Autodesk Fusion 360 part; units mm, degrees
note: some values were not read from the file. Set by a fixed rule: which sketch regions a step uses.
(part 3 of 6)
  line L1897 (389.5, 225.3453) -> (391.5, 224.1906)
  line L1898 (364.75, 196.4178) -> (364.75, 194.1084)
  line L1899 (377.75, 201.9537) -> (379.75, 203.1084)
  line L1900 (381.25, 203.1084) -> (383.25, 201.9537)
  line L1901 (386.75, 230.1084) -> (388.75, 228.9537)
  line L1902 (355, 207.3453) -> (355, 209.6547)
  line L1903 (381.25, 205.4178) -> (381.25, 203.1084)
  line L1904 (366.75, 197.5725) -> (364.75, 196.4178)
  line L1905 (399.75, 237.9537) -> (401.75, 239.1084)
  line L1906 (363.25, 212.1084) -> (363.25, 214.4178)
  line L1907 (390.75, 221.1084) -> (390.75, 223.4178)
  line L1908 (377, 198.3453) -> (377, 200.6547)
  line L1909 (369.5, 233.1906) -> (371.5, 234.3453)
  line L1910 (361.25, 206.5725) -> (359.25, 205.4178)
  line L1911 (388, 225.3453) -> (388, 227.6547)
  line L1912 (362, 198.3453) -> (364, 197.1906)
  line L1913 (368.75, 194.1084) -> (368.75, 196.4178)
  line L1914 (385.25, 221.1084) -> (385.25, 223.4178)
  line L1915 (364.75, 214.4178) -> (364.75, 212.1084)
  line L1916 (389.5, 225.3453) -> (391.5, 224.1906)
  line L1917 (371.5, 227.6547) -> (369.5, 228.8094)
  line L1918 (356.5, 207.3453) -> (358.5, 206.1906)
  line L1919 (366, 191.6547) -> (364, 192.8094)
  line L1920 (364.75, 203.1084) -> (366.75, 201.9537)
  line L1921 (364, 197.1906) -> (366, 198.3453)
  line L1922 (399, 234.3453) -> (399, 236.6547)
  line L1923 (353.75, 212.1084) -> (355.75, 210.9537)
  line L1924 (358.5, 210.8094) -> (356.5, 209.6547)
  line L1925 (366, 200.6547) -> (364, 201.8094)
  line L1926 (393.5, 234.3453) -> (393.5, 236.6547)
  line L1927 (358.5, 206.1906) -> (360.5, 207.3453)
  line L1928 (384, 225.3453) -> (386, 224.1906)
  line L1929 (364.75, 194.1084) -> (366.75, 192.9537)
  line L1930 (371.5, 236.6547) -> (369.5, 237.8094)
  line L1931 (381.25, 241.4178) -> (381.25, 239.1084)
  line L1932 (357.75, 205.4178) -> (355.75, 206.5725)
  line L1933 (373, 252.3453) -> (375, 251.1906)
  line L1934 (381.25, 196.4178) -> (381.25, 194.1084)
  line L1935 (364, 192.8094) -> (362, 191.6547)
  line L1936 (372.25, 251.5725) -> (370.25, 250.4178)
  line L1937 (355.75, 210.9537) -> (357.75, 212.1084)
  line L1938 (372.25, 242.5725) -> (370.25, 241.4178)
  line L1939 (380.5, 201.8094) -> (378.5, 200.6547)
  line L1940 (393.5, 234.3453) -> (393.5, 236.6547)
  line L1941 (369.5, 242.1906) -> (371.5, 243.3453)
  line L1942 (392.25, 241.4178) -> (392.25, 239.1084)
  line L1943 (372.25, 251.5725) -> (370.25, 250.4178)
  line L1944 (357.75, 221.1084) -> (357.75, 223.4178)
  line L1945 (386.75, 223.4178) -> (386.75, 221.1084)
  line L1946 (388.75, 224.5725) -> (386.75, 223.4178)
  line L1947 (366, 198.3453) -> (366, 200.6547)
  line L1948 (355.75, 210.9537) -> (357.75, 212.1084)
  line L1949 (375.75, 203.1084) -> (377.75, 201.9537)
  line L1950 (368.75, 196.4178) -> (366.75, 197.5725)
  line L1951 (386, 228.8094) -> (384, 227.6547)
  line L1952 (384, 227.6547) -> (384, 225.3453)
  line L1953 (383.25, 215.5725) -> (381.25, 214.4178)
  line L1954 (390.75, 223.4178) -> (388.75, 224.5725)
  line L1955 (375, 237.8094) -> (373, 236.6547)
  line L1956 (381.25, 194.1084) -> (383.25, 192.9537)
  line L1957 (357.75, 205.4178) -> (355.75, 206.5725)
  line L1958 (402.5, 237.8094) -> (400.5, 236.6547)
  line L1959 (374.25, 248.1084) -> (374.25, 250.4178)
  line L1960 (371.5, 236.6547) -> (369.5, 237.8094)
  line L1961 (356.5, 209.6547) -> (356.5, 207.3453)
  line L1962 (380.5, 197.1906) -> (382.5, 198.3453)
  line L1963 (379.75, 194.1084) -> (379.75, 196.4178)
  line L1964 (370.25, 241.4178) -> (370.25, 239.1084)
  line L1965 (404.5, 227.6547) -> (402.5, 228.8094)
  line L1966 (400.5, 236.6547) -> (400.5, 234.3453)
  line L1967 (402.5, 237.8094) -> (400.5, 236.6547)
  line L1968 (371.5, 243.3453) -> (371.5, 245.6547)
  line L1969 (356.5, 209.6547) -> (356.5, 207.3453)
  line L1970 (382.5, 198.3453) -> (382.5, 200.6547)
  line L1971 (362, 198.3453) -> (364, 197.1906)
  line L1972 (381.25, 196.4178) -> (381.25, 194.1084)
  line L1973 (386, 224.1906) -> (388, 225.3453)
  line L1974 (395, 236.6547) -> (395, 234.3453)
  line L1975 (382.5, 200.6547) -> (380.5, 201.8094)
  line L1976 (355.75, 206.5725) -> (353.75, 205.4178)
  line L1977 (377.75, 192.9537) -> (379.75, 194.1084)
  line L1978 (353.75, 223.4178) -> (353.75, 221.1084)
  line L1979 (364.75, 194.1084) -> (366.75, 192.9537)
  line L1980 (389.5, 227.6547) -> (389.5, 225.3453)
  line L1981 (400.5, 234.3453) -> (402.5, 233.1906)
  line L1982 (400.5, 236.6547) -> (400.5, 234.3453)
  line L1983 (374.25, 241.4178) -> (372.25, 242.5725)
  line L1984 (381.25, 212.1084) -> (383.25, 210.9537)
  line L1985 (370.25, 250.4178) -> (370.25, 248.1084)
  line L1986 (369.5, 233.1906) -> (371.5, 234.3453)
  line L1987 (395, 236.6547) -> (395, 234.3453)
  line L1988 (375.75, 194.1084) -> (377.75, 192.9537)
  line L1989 (383.25, 206.5725) -> (381.25, 205.4178)
  line L1990 (352.25, 221.1084) -> (352.25, 223.4178)
  line L1991 (346.75, 221.1084) -> (346.75, 223.4178)
  line L1992 (375.75, 241.4178) -> (375.75, 239.1084)
  line L1993 (346.75, 221.1084) -> (346.75, 223.4178)
  line L1994 (370.25, 250.4178) -> (370.25, 248.1084)
  line L1995 (356.5, 216.3453) -> (358.5, 215.1906)
  line L1996 (378.5, 200.6547) -> (378.5, 198.3453)
  line L1997 (385.25, 205.4178) -> (383.25, 206.5725)
  line L1998 (370.25, 248.1084) -> (372.25, 246.9537)
  line L1999 (372.25, 246.9537) -> (374.25, 248.1084)
  line L2000 (369.5, 251.1906) -> (371.4564, 252.3202)
  line L2001 (388.75, 206.5725) -> (386.75, 205.4178)
  line L2002 (379.75, 196.4178) -> (377.75, 197.5725)
  line L2003 (390.75, 205.4178) -> (388.75, 206.5725)
  line L2004 (375, 237.8094) -> (373, 236.6547)
  line L2005 (353, 215.1906) -> (355, 216.3453)
  line L2006 (348.25, 223.4178) -> (348.25, 221.1084)
  line L2007 (386, 210.8094) -> (384, 209.6547)
  line L2008 (372.25, 237.9537) -> (374.25, 239.1084)
  line L2009 (355, 218.6547) -> (353, 219.8094)
  line L2010 (371.5, 218.6547) -> (369.5, 219.8094)
  line L2011 (384, 209.6547) -> (384, 207.3453)
  line L2012 (369.5, 251.1906) -> (371.4564, 252.3202)
  line L2013 (385.25, 196.4178) -> (383.25, 197.5725)
  line L2014 (361.25, 215.5725) -> (359.25, 214.4178)
  line L2015 (381.25, 203.1084) -> (383.25, 201.9537)
  line L2016 (375, 246.8094) -> (373, 245.6547)
  line L2017 (372.25, 237.9537) -> (374.25, 239.1084)
  line L2018 (374.25, 239.1084) -> (374.25, 241.4178)
  line L2019 (355.75, 215.5725) -> (353.75, 214.4178)
  line L2020 (383.25, 201.9537) -> (385.25, 203.1084)
  line L2021 (385.25, 214.4178) -> (383.25, 215.5725)
  line L2022 (381.25, 194.1084) -> (383.25, 192.9537)
  line L2023 (380.5, 201.8094) -> (378.5, 200.6547)
  line L2024 (382.5, 225.3453) -> (382.5, 227.6547)
  line L2025 (352.25, 239.1084) -> (352.25, 241.4178)
  line L2026 (357.75, 214.4178) -> (355.75, 215.5725)
  line L2027 (389.5, 209.6547) -> (389.5, 207.3453)
  line L2028 (370.25, 248.1084) -> (372.25, 246.9537)
  line L2029 (373, 252.4428) -> (373, 252.3453)
  line L2030 (385.25, 214.4178) -> (383.25, 215.5725)
  line L2031 (375.75, 194.1084) -> (377.75, 192.9537)
  line L2032 (383.25, 210.9537) -> (385.25, 212.1084)
  line L2033 (386.75, 212.1084) -> (388.75, 210.9537)
  line L2034 (383.25, 206.5725) -> (381.25, 205.4178)
  line L2035 (388, 207.3453) -> (388, 209.6547)
  line L2036 (382.5, 198.3453) -> (382.5, 200.6547)
  line L2037 (375.75, 223.4178) -> (375.75, 221.1084)
  line L2038 (383.25, 197.5725) -> (381.25, 196.4178)
  line L2039 (383.25, 197.5725) -> (381.25, 196.4178)
  line L2040 (377.75, 228.9537) -> (379.75, 230.1084)
  line L2041 (381.25, 223.4178) -> (381.25, 221.1084)
  line L2042 (383.25, 192.9537) -> (385.25, 194.1084)
  line L2043 (377.75, 197.5725) -> (375.75, 196.4178)
  line L2044 (381.25, 212.1084) -> (383.25, 210.9537)
  line L2045 (355, 216.3453) -> (355, 218.6547)
  line L2046 (383.25, 210.9537) -> (385.25, 212.1084)
  line L2047 (359.25, 223.4178) -> (359.25, 221.1084)
  line L2048 (388, 207.3453) -> (388, 209.6547)
  line L2049 (353, 215.1906) -> (355, 216.3453)
  line L2050 (360.5, 218.6547) -> (358.5, 219.8094)
  line L2051 (390.75, 205.4178) -> (388.75, 206.5725)
  arc A62 (371.4564, 252.3202) -> (368.3398, 251.8605) centre (375, 217.5) ccw
  line L2052 (388, 209.6547) -> (386, 210.8094)
  line L2053 (369.5, 224.1906) -> (371.5, 225.3453)
  line L2054 (373, 245.6547) -> (373, 243.3453)
  line L2055 (380.5, 197.1906) -> (382.5, 198.3453)
  line L2056 (382.5, 225.3453) -> (382.5, 227.6547)
  line L2057 (389.5, 209.6547) -> (389.5, 207.3453)
  line L2058 (373, 243.3453) -> (375, 242.1906)
  line L2059 (383.25, 192.9537) -> (385.25, 194.1084)
  line L2060 (358.5, 219.8094) -> (356.5, 218.6547)
  line L2061 (360.5, 216.3453) -> (360.5, 218.6547)
  line L2062 (358.5, 215.1906) -> (360.5, 216.3453)
  line L2063 (370.25, 239.1084) -> (372.25, 237.9537)
  line L2064 (375.75, 223.4178) -> (375.75, 221.1084)
  line L2065 (371.5, 243.3453) -> (371.5, 245.6547)
  line L2066 (389.5, 207.3453) -> (391.5, 206.1906)
  line L2067 (375.75, 230.1084) -> (377.75, 228.9537)
  line L2068 (388.75, 210.9537) -> (390.75, 212.1084)
  line L2069 (386, 206.1906) -> (388, 207.3453)
  line L2070 (379.75, 221.1084) -> (379.75, 223.4178)
  line L2071 (378.5, 227.6547) -> (378.5, 225.3453)
  line L2072 (374.25, 248.1084) -> (374.25, 250.4178)
  line L2073 (386.75, 232.4178) -> (386.75, 230.1084)
  line L2074 (389.5, 207.3453) -> (391.5, 206.1906)
  line L2075 (370.25, 239.1084) -> (372.25, 237.9537)
  line L2076 (362, 218.6547) -> (362, 216.3453)
  line L2077 (384, 209.6547) -> (384, 207.3453)
  line L2078 (360.5, 218.6547) -> (358.5, 219.8094)
  line L2079 (379.75, 248.1084) -> (379.75, 250.4178)
  line L2080 (369.5, 215.1906) -> (371.5, 216.3453)
  line L2081 (358.5, 219.8094) -> (356.5, 218.6547)
  line L2082 (377, 225.3453) -> (377, 227.6547)
  line L2083 (388.75, 206.5725) -> (386.75, 205.4178)
  line L2084 (360.5, 225.3453) -> (360.5, 227.6547)
  line L2085 (391.5, 210.8094) -> (389.5, 209.6547)
  line L2086 (383.25, 215.5725) -> (381.25, 214.4178)
  line L2087 (372.25, 246.9537) -> (374.25, 248.1084)
  line L2088 (371.5, 227.6547) -> (369.5, 228.8094)
  line L2089 (355, 209.6547) -> (353, 210.8094)
  line L2090 (359.25, 241.4178) -> (359.25, 239.1084)
  line L2091 (391.5, 210.8094) -> (389.5, 209.6547)
  line L2092 (374.25, 250.4178) -> (372.25, 251.5725)
  line L2093 (377.75, 224.5725) -> (375.75, 223.4178)
  line L2094 (386, 206.1906) -> (388, 207.3453)
  line L2095 (348.25, 240.0707) -> (348.25, 239.1084)
  line L2096 (374.25, 239.1084) -> (374.25, 241.4178)
  line L2097 (381.25, 223.4178) -> (381.25, 221.1084)
  line L2098 (385.25, 205.4178) -> (383.25, 206.5725)
  line L2099 (373, 252.4428) -> (373, 252.3453)
  line L2100 (380.5, 224.1906) -> (382.5, 225.3453)
  line L2101 (355.75, 228.9537) -> (357.75, 230.1084)
  line L2102 (382.5, 227.6547) -> (380.5, 228.8094)
  line L2103 (355.75, 215.5725) -> (353.75, 214.4178)
  line L2104 (369.5, 242.1906) -> (371.5, 243.3453)
  line L2105 (371.5, 218.6547) -> (369.5, 219.8094)
  line L2106 (369.5, 215.1906) -> (371.5, 216.3453)
  line L2107 (353.75, 221.1084) -> (355.75, 219.9537)
  line L2108 (373, 243.3453) -> (375, 242.1906)
  line L2109 (379.75, 221.1084) -> (379.75, 223.4178)
  line L2110 (357.75, 239.1084) -> (357.75, 241.4178)
  line L2111 (358.5, 215.1906) -> (360.5, 216.3453)
  line L2112 (383.25, 201.9537) -> (385.25, 203.1084)
  line L2113 (390.75, 212.1084) -> (390.75, 214.4178)
  line L2114 (385.25, 196.4178) -> (383.25, 197.5725)
  line L2115 (373, 245.6547) -> (373, 243.3453)
  line L2116 (356.5, 227.6547) -> (356.5, 225.3453)
  line L2117 (353, 206.1906) -> (355, 207.3453)
  line L2118 (355, 216.3453) -> (355, 218.6547)
  line L2119 (384, 207.3453) -> (386, 206.1906)
  line L2120 (377, 225.3453) -> (377, 227.6547)
  line L2121 (382.5, 209.6547) -> (380.5, 210.8094)
  line L2122 (388, 209.6547) -> (386, 210.8094)
  line L2123 (373, 236.6547) -> (373, 234.3453)
  line L2124 (388, 245.6547) -> (386, 246.8094)
  line L2125 (360.5, 216.3453) -> (360.5, 218.6547)
  line L2126 (372.25, 242.5725) -> (370.25, 241.4178)
  line L2127 (379.75, 230.1084) -> (379.75, 232.4178)
  line L2128 (359.25, 221.1084) -> (361.25, 219.9537)
  line L2129 (357.75, 223.4178) -> (355.75, 224.5725)
  line L2130 (392.25, 214.4178) -> (392.25, 212.1084)
  line L2131 (375, 246.8094) -> (373, 245.6547)
  line L2132 (356.5, 225.3453) -> (358.5, 224.1906)
  line L2133 (362, 227.6547) -> (362, 225.3453)
  line L2134 (373, 252.3453) -> (375, 251.1906)
  line L2135 (362, 227.6547) -> (362, 225.3453)
  line L2136 (355.75, 219.9537) -> (357.75, 221.1084)
  line L2137 (375.75, 230.1084) -> (377.75, 228.9537)
  line L2138 (378.5, 207.3453) -> (380.5, 206.1906)
  line L2139 (356.5, 225.3453) -> (358.5, 224.1906)
  line L2140 (382.5, 209.6547) -> (380.5, 210.8094)
  line L2141 (386, 210.8094) -> (384, 209.6547)
  line L2142 (359.25, 230.1084) -> (361.25, 228.9537)
  line L2143 (392.25, 214.4178) -> (392.25, 212.1084)
  line L2144 (384, 207.3453) -> (386, 206.1906)
  line L2145 (386.75, 248.1084) -> (388.75, 246.9537)
  line L2146 (378.5, 225.3453) -> (380.5, 224.1906)
  line L2147 (359.25, 230.1084) -> (361.25, 228.9537)
  line L2148 (385.25, 212.1084) -> (385.25, 214.4178)
  line L2149 (386, 246.8094) -> (384, 245.6547)
  line L2150 (377, 207.3453) -> (377, 209.6547)
  line L2151 (371.5, 234.3453) -> (371.5, 236.6547)
  line L2152 (380.5, 224.1906) -> (382.5, 225.3453)
  line L2153 (379.75, 223.4178) -> (377.75, 224.5725)
  line L2154 (374.25, 250.4178) -> (372.25, 251.5725)
  line L2155 (357.75, 214.4178) -> (355.75, 215.5725)
  line L2156 (379.75, 230.1084) -> (379.75, 232.4178)
  line L2157 (359.25, 221.1084) -> (361.25, 219.9537)
  line L2158 (386.75, 212.1084) -> (388.75, 210.9537)
  line L2159 (361.25, 224.5725) -> (359.25, 223.4178)
  line L2160 (389.5, 243.3453) -> (391.5, 242.1906)
  line L2161 (380.5, 228.8094) -> (378.5, 227.6547)
  line L2162 (357.75, 223.4178) -> (355.75, 224.5725)
  line L2163 (390.75, 212.1084) -> (390.75, 214.4178)
  line L2164 (361.25, 215.5725) -> (359.25, 214.4178)
  line L2165 (375.75, 250.4178) -> (375.75, 248.1084)
  line L2166 (374.25, 241.4178) -> (372.25, 242.5725)
  line L2167 (375.75, 212.1084) -> (377.75, 210.9537)
  line L2168 (370.25, 241.4178) -> (370.25, 239.1084)
  line L2169 (382.5, 227.6547) -> (380.5, 228.8094)
  line L2170 (377.75, 228.9537) -> (379.75, 230.1084)
  line L2171 (388.75, 210.9537) -> (390.75, 212.1084)
  line L2172 (356.5, 218.6547) -> (356.5, 216.3453)
  line L2173 (362, 218.6547) -> (362, 216.3453)
  line L2174 (373, 236.6547) -> (373, 234.3453)
  line L2175 (377.75, 206.5725) -> (375.75, 205.4178)
  line L2176 (379.75, 223.4178) -> (377.75, 224.5725)
  line L2177 (378.5, 225.3453) -> (380.5, 224.1906)
  line L2178 (356.5, 218.6547) -> (356.5, 216.3453)
  line L2179 (361.25, 224.5725) -> (359.25, 223.4178)
  arc A63 (371.4564, 252.3202) -> (368.3398, 251.8605) centre (375, 217.5) ccw
  line L2180 (379.75, 205.4178) -> (377.75, 206.5725)
  line L2181 (380.5, 228.8094) -> (378.5, 227.6547)
  line L2182 (355.75, 219.9537) -> (357.75, 221.1084)
  line L2183 (360.5, 227.6547) -> (358.5, 228.8094)
  line L2184 (377.75, 224.5725) -> (375.75, 223.4178)
  line L2185 (382.5, 207.3453) -> (382.5, 209.6547)
  line L2186 (353.75, 241.4178) -> (353.75, 239.1084)
  line L2187 (356.5, 216.3453) -> (358.5, 215.1906)
  line L2188 (388.75, 242.5725) -> (386.75, 241.4178)
  line L2189 (389.5, 245.6547) -> (389.5, 243.3453)
  line L2190 (371.5, 234.3453) -> (371.5, 236.6547)
  line L2191 (353.75, 230.1084) -> (355.75, 228.9537)
  arc A64 (387.3612, 184.7555) -> (390.75, 186.244) centre (375, 217.5) ccw
  arc A65 (387.3612, 184.7555) -> (390.75, 186.244) centre (375, 217.5) ccw
  line L2192 (388.75, 188.5725) -> (386.75, 187.4178)
  line L2193 (390.75, 187.4178) -> (388.75, 188.5725)
  line L2194 (384, 189.3453) -> (386, 188.1906)
  line L2195 (388, 189.3453) -> (388, 191.6547)
  line L2196 (380.5, 188.1906) -> (382.5, 189.3453)
  line L2197 (381.25, 187.4178) -> (381.25, 185.1084)
  line L2198 (386.75, 187.4178) -> (386.75, 185.1084)
  line L2199 (380.5, 188.1906) -> (382.5, 189.3453)
  line L2200 (375.75, 187.4178) -> (375.75, 185.1084)
  line L2201 (386, 188.1906) -> (388, 189.3453)
  line L2202 (379.75, 187.4178) -> (377.75, 188.5725)
  line L2203 (379.75, 185.1084) -> (379.75, 187.4178)
  line L2204 (386.75, 187.4178) -> (386.75, 185.1084)
  line L2205 (375.75, 187.4178) -> (375.75, 185.1084)
  line L2206 (381.25, 187.4178) -> (381.25, 185.1084)
  line L2207 (388.75, 188.5725) -> (386.75, 187.4178)
  line L2208 (379.75, 185.1084) -> (379.75, 187.4178)
  line L2209 (385.25, 185.1084) -> (385.25, 187.4178)
  line L2210 (375, 233.1906) -> (377, 234.3453)
  line L2211 (390.75, 187.4178) -> (388.75, 188.5725)
  line L2212 (385.25, 185.1084) -> (385.25, 187.4178)
  line L2213 (402.5, 197.1906) -> (404.1665, 198.1527)
  line L2214 (400.5, 198.3453) -> (402.5, 197.1906)
  line L2215 (404.5, 200.6547) -> (402.5, 201.8094)
  line L2216 (402.5, 206.1906) -> (404.5, 207.3453)
  line L2217 (400.5, 198.3453) -> (402.5, 197.1906)
  line L2218 (402.5, 201.8094) -> (400.5, 200.6547)
  line L2219 (404.5, 200.6547) -> (402.5, 201.8094)
  line L2220 (400.5, 207.3453) -> (402.5, 206.1906)
  line L2221 (395, 200.6547) -> (395, 198.3453)
  line L2222 (399, 198.3453) -> (399, 200.6547)
  line L2223 (395, 200.6547) -> (395, 198.3453)
  line L2224 (393.5, 198.3453) -> (393.5, 200.6547)
  line L2225 (400.5, 200.6547) -> (400.5, 198.3453)
  line L2226 (402.5, 201.8094) -> (400.5, 200.6547)
  line L2227 (393.5, 198.3453) -> (393.5, 200.6547)
  line L2228 (402.5, 206.1906) -> (404.5, 207.3453)
  line L2229 (400.5, 200.6547) -> (400.5, 198.3453)
  line L2230 (391.5, 188.1906) -> (393.5, 189.3453)
  line L2231 (389.5, 189.3453) -> (391.5, 188.1906)
  line L2232 (393.5, 189.3453) -> (393.5, 191.6547)
  line L2233 (390.75, 186.244) -> (390.75, 187.4178)
  line L2234 (393.5, 189.3453) -> (393.5, 191.6547)
  line L2235 (392.25, 187.4178) -> (392.25, 187.0461)
  line L2236 (391.5, 188.1906) -> (393.5, 189.3453)
  line L2237 (390.75, 186.244) -> (390.75, 187.4178)
  line L2238 (389.5, 189.3453) -> (391.5, 188.1906)
  line L2239 (389.5, 191.6547) -> (389.5, 189.3453)
  line L2240 (392.25, 187.4178) -> (392.25, 187.0461)
  line L2241 (399.75, 206.5725) -> (397.75, 205.4178)
  line L2242 (399.75, 201.9537) -> (401.75, 203.1084)
  line L2243 (397, 201.8094) -> (395, 200.6547)
  line L2244 (395, 207.3453) -> (397, 206.1906)
  line L2245 (394.25, 201.9537) -> (396.25, 203.1084)
  line L2246 (395, 207.3453) -> (397, 206.1906)
  line L2247 (397.75, 205.4178) -> (397.75, 203.1084)
  line L2248 (401.75, 203.1084) -> (401.75, 205.4178)
  line L2249 (396.25, 203.1084) -> (396.25, 205.4178)
  line L2250 (397, 206.1906) -> (399, 207.3453)
  line L2251 (401.75, 205.4178) -> (399.75, 206.5725)
  line L2252 (397, 206.1906) -> (399, 207.3453)
  line L2253 (397.75, 205.4178) -> (397.75, 203.1084)
  line L2254 (397.75, 203.1084) -> (399.75, 201.9537)
  line L2255 (397, 201.8094) -> (395, 200.6547)
  line L2256 (399, 198.3453) -> (399, 200.6547)
  line L2257 (399, 200.6547) -> (397, 201.8094)
  line L2258 (399.75, 206.5725) -> (397.75, 205.4178)
  line L2259 (399.75, 201.9537) -> (401.75, 203.1084)
  line L2260 (396.25, 205.4178) -> (394.25, 206.5725)
  line L2261 (394.25, 201.9537) -> (396.25, 203.1084)
  line L2262 (405.25, 206.5725) -> (403.25, 205.4178)
  line L2263 (405.25, 206.5725) -> (403.25, 205.4178)
  line L2264 (403.25, 203.1084) -> (405.25, 201.9537)
  line L2265 (403.25, 205.4178) -> (403.25, 203.1084)
  line L2266 (407.25, 205.4178) -> (405.25, 206.5725)
  arc A66 (406.7807, 202.8375) -> (407.25, 203.9008) centre (375, 217.5) ccw
  arc A67 (406.7807, 202.8375) -> (407.25, 203.9008) centre (375, 217.5) ccw
  line L2267 (405.25, 201.9537) -> (406.7807, 202.8375)
  line L2268 (408, 206.1906) -> (408.1524, 206.2786)
  line L2269 (407.25, 203.9008) -> (407.25, 205.4178)
  arc A68 (404.1665, 198.1527) -> (404.5, 198.6652) centre (375, 217.5) ccw
  line L2270 (403.25, 205.4178) -> (403.25, 203.1084)
  line L2271 (406, 207.3453) -> (408, 206.1906)
  line L2272 (403.25, 203.1084) -> (405.25, 201.9537)
  arc A69 (404.1665, 198.1527) -> (404.5, 198.6652) centre (375, 217.5) ccw
  line L2273 (405.25, 201.9537) -> (406.7807, 202.8375)
  line L2274 (407.25, 205.4178) -> (405.25, 206.5725)
  line L2275 (408, 206.1906) -> (408.1524, 206.2786)
  line L2276 (404.5, 198.6652) -> (404.5, 200.6547)
  line L2277 (406, 207.3453) -> (408, 206.1906)
  line L2278 (404.5, 198.6652) -> (404.5, 200.6547)
  line L2279 (407.25, 203.9008) -> (407.25, 205.4178)
  line L2280 (396.25, -88.5822) -> (394.25, -87.4275)
  line L2281 (397.75, -90.8916) -> (399.75, -92.0463)
  line L2282 (401.75, -90.8916) -> (401.75, -88.5822)
  line L2283 (399, -93.3453) -> (397, -92.1906)
  line L2284 (396.25, -90.8916) -> (396.25, -88.5822)
  line L2285 (401.75, -88.5822) -> (399.75, -87.4275)
  line L2286 (395, -95.6547) -> (397, -96.8094)
  line L2287 (401.75, -97.5822) -> (399.75, -96.4275)
  line L2288 (397.75, -97.5822) -> (397.75, -99.8916)
  line L2289 (397.75, -97.5822) -> (397.75, -99.8916)
  arc A70 (400.2057, -100.7831) -> (401.75, -99.0707) centre (375, -76.5) ccw
  line L2290 (397, -96.8094) -> (399, -95.6547)
  line L2291 (397.75, -99.8916) -> (399.75, -101.0463)
  line L2292 (396.25, -97.5822) -> (394.25, -96.4275)
  line L2293 (396.25, -97.5822) -> (394.25, -96.4275)
  line L2294 (401.75, -99.0707) -> (401.75, -97.5822)
  line L2295 (399.75, -101.0463) -> (400.2057, -100.7831)
  arc A71 (400.2057, -100.7831) -> (401.75, -99.0707) centre (375, -76.5) ccw
  line L2296 (396.25, -99.8916) -> (396.25, -97.5822)
  line L2297 (396.25, -99.8916) -> (396.25, -97.5822)
  line L2298 (401.75, -97.5822) -> (399.75, -96.4275)
  line L2299 (397.75, -99.8916) -> (399.75, -101.0463)
  line L2300 (399.75, -101.0463) -> (400.2057, -100.7831)
  line L2301 (399.75, -96.4275) -> (397.75, -97.5822)
  line L2302 (401.75, -99.0707) -> (401.75, -97.5822)
  line L2303 (395, -95.6547) -> (397, -96.8094)
  line L2304 (399.75, -96.4275) -> (397.75, -97.5822)
  line L2305 (397, -96.8094) -> (399, -95.6547)
  line L2306 (394.25, -101.0463) -> (396.25, -99.8916)
  line L2307 (394.25, -101.0463) -> (396.25, -99.8916)
  line L2308 (375, -105.8094) -> (377, -104.6547)
  line L2309 (389.5, -102.3453) -> (389.5, -104.6547)
  arc A72 (395.442, -104.9099) -> (398.7552, -102.2039) centre (375, -76.5) ccw
  line L2310 (395, -104.6547) -> (395.442, -104.9099)
  line L2311 (395, -102.3453) -> (395, -104.6547)
  arc A73 (395.442, -104.9099) -> (398.7552, -102.2039) centre (375, -76.5) ccw
  line L2312 (395, -102.3453) -> (395, -104.6547)
  line L2313 (395, -104.6547) -> (395.442, -104.9099)
  line L2314 (396.25, -81.8916) -> (396.25, -79.5822)
  line L2315 (397.75, -79.5822) -> (397.75, -81.8916)
  line L2316 (377, -57.3453) -> (375, -56.1906)
  line L2317 (395, -77.6547) -> (397, -78.8094)
  line L2318 (399.75, -83.0463) -> (401.75, -81.8916)
  line L2319 (375, -87.8094) -> (377, -86.6547)
  line L2320 (399, -84.3453) -> (397, -83.1906)
  line L2321 (397.75, -81.8916) -> (399.75, -83.0463)
  line L2322 (399, -84.3453) -> (397, -83.1906)
  line L2323 (397.75, -81.8916) -> (399.75, -83.0463)
  line L2324 (396.25, -79.5822) -> (394.25, -78.4275)
  line L2325 (375, -96.8094) -> (377, -95.6547)
  line L2326 (397.75, -79.5822) -> (397.75, -81.8916)
  line L2327 (375, -87.8094) -> (377, -86.6547)
  line L2328 (401.75, -81.8916) -> (401.75, -79.5822)
  line L2329 (375, -69.8094) -> (377, -68.6547)
  line L2330 (394.25, -83.0463) -> (396.25, -81.8916)
  arc A74 (377, -41.5572) -> (373, -41.5572) centre (375, -76.5) ccw
  line L2331 (375, -78.8094) -> (377, -77.6547)
  line L2332 (377, -84.3453) -> (375, -83.1906)
  line L2333 (375, -60.8094) -> (377, -59.6547)
  line L2334 (399.75, -83.0463) -> (401.75, -81.8916)
  line L2335 (377, -111.3453) -> (375, -110.1906)
  line L2336 (375, -78.8094) -> (377, -77.6547)
  line L2337 (375, -42.8094) -> (377, -41.6547)
  line L2338 (401.75, -79.5822) -> (399.75, -78.4275)
  line L2339 (395, -77.6547) -> (397, -78.8094)
  line L2340 (377, -48.3453) -> (375, -47.1906)
  line L2341 (401.75, -79.5822) -> (399.75, -78.4275)
  line L2342 (396.25, -79.5822) -> (394.25, -78.4275)
  line L2343 (396.25, -81.8916) -> (396.25, -79.5822)
  line L2344 (375, -105.8094) -> (377, -104.6547)
  line L2345 (375, -69.8094) -> (377, -68.6547)
  line L2346 (377, -93.3453) -> (375, -92.1906)
  line L2347 (375, -42.8094) -> (377, -41.6547)
  line L2348 (397, -78.8094) -> (399, -77.6547)
  line L2349 (377, -102.3453) -> (375, -101.1906)
  line L2350 (377, -111.3453) -> (375, -110.1906)
  line L2351 (377, -57.3453) -> (375, -56.1906)
  line L2352 (397, -83.1906) -> (395, -84.3453)
  line L2353 (377, -66.3453) -> (375, -65.1906)
  line L2354 (375, -96.8094) -> (377, -95.6547)
  line L2355 (377, -93.3453) -> (375, -92.1906)
  line L2356 (377, -84.3453) -> (375, -83.1906)
  line L2357 (398.7552, -102.2039) -> (397, -101.1906)
  line L2358 (377, -102.3453) -> (375, -101.1906)
  line L2359 (401.75, -70.5822) -> (399.75, -69.4275)
  line L2360 (394.25, -96.4275) -> (392.25, -97.5822)
  arc A75 (342.75, -90.0992) -> (343.2193, -91.1625) centre (375, -76.5) ccw
  line L2361 (391.5, -78.8094) -> (393.5, -77.6547)
  line L2362 (348.25, -88.5822) -> (348.25, -90.8916)
  line L2363 (386, -101.1906) -> (384, -102.3453)
  line L2364 (368.75, -90.8916) -> (368.75, -88.5822)
  line L2365 (375, -51.8094) -> (377, -50.6547)
  line L2366 (353.75, -88.5822) -> (353.75, -90.8916)
  line L2367 (377, -66.3453) -> (375, -65.1906)
  line L2368 (399.75, -78.4275) -> (397.75, -79.5822)
  line L2369 (380.5, -101.1906) -> (378.5, -102.3453)
  line L2370 (377, -75.3453) -> (375, -74.1906)
  line L2371 (397, -78.8094) -> (399, -77.6547)
  line L2372 (346.75, -90.8916) -> (346.75, -88.5822)
  line L2373 (386, -101.1906) -> (384, -102.3453)
  line L2374 (382.5, -102.3453) -> (380.5, -101.1906)
  line L2375 (399.75, -78.4275) -> (397.75, -79.5822)
  line L2376 (391.5, -101.1906) -> (389.5, -102.3453)
  arc A76 (342.75, -90.0992) -> (343.2193, -91.1625) centre (375, -76.5) ccw
  line L2377 (363.25, -90.8916) -> (363.25, -88.5822)
  line L2378 (348.25, -88.5822) -> (348.25, -90.8916)
  line L2379 (359.25, -88.5822) -> (359.25, -90.8916)
  line L2380 (394.25, -83.0463) -> (396.25, -81.8916)
  line L2381 (353.75, -88.5822) -> (353.75, -90.8916)
  line L2382 (397, -101.1906) -> (395, -102.3453)
  line L2383 (377, -48.3453) -> (375, -47.1906)
  line L2384 (352.25, -90.8916) -> (352.25, -88.5822)
  line L2385 (393.5, -102.3453) -> (391.5, -101.1906)
  line L2386 (391.5, -101.1906) -> (389.5, -102.3453)
  line L2387 (382.5, -102.3453) -> (380.5, -101.1906)
  line L2388 (395, -68.6547) -> (397, -69.8094)
  line L2389 (399, -75.3453) -> (397, -74.1906)
  line L2390 (398.7552, -102.2039) -> (397, -101.1906)
  line L2391 (397, -83.1906) -> (395, -84.3453)
  line L2392 (388, -102.3453) -> (386, -101.1906)
  line L2393 (401.75, -81.8916) -> (401.75, -79.5822)
  line L2394 (380.5, -101.1906) -> (378.5, -102.3453)
  arc A77 (373, -111.4428) -> (377, -111.4428) centre (375, -76.5) ccw
  line L2395 (396.25, -72.8916) -> (396.25, -70.5822)
  line L2396 (357.75, -90.8916) -> (357.75, -88.5822)
  line L2397 (377, -75.3453) -> (375, -74.1906)
  line L2398 (357.75, -90.8916) -> (357.75, -88.5822)
  line L2399 (397, -101.1906) -> (395, -102.3453)
  line L2400 (346.75, -90.8916) -> (346.75, -88.5822)
  line L2401 (399, -75.3453) -> (397, -74.1906)
  line L2402 (374.25, -90.8916) -> (374.25, -88.5822)
  line L2403 (397, -74.1906) -> (395, -75.3453)
  line L2404 (370.25, -88.5822) -> (370.25, -90.8916)
  line L2405 (364.75, -88.5822) -> (364.75, -90.8916)
  line L2406 (396.25, -72.8916) -> (396.25, -70.5822)
  line L2407 (359.25, -88.5822) -> (359.25, -90.8916)
  arc A78 (373, -111.4428) -> (377, -111.4428) centre (375, -76.5) ccw
  line L2408 (393.5, -102.3453) -> (391.5, -101.1906)
  line L2409 (388, -102.3453) -> (386, -101.1906)
  line L2410 (352.25, -90.8916) -> (352.25, -88.5822)
  line L2411 (364.75, -88.5822) -> (364.75, -90.8916)
  line L2412 (368.75, -90.8916) -> (368.75, -88.5822)
  line L2413 (397.75, -70.5822) -> (397.75, -72.8916)
  line L2414 (363.25, -90.8916) -> (363.25, -88.5822)
  line L2415 (401.75, -70.5822) -> (399.75, -69.4275)
  line L2416 (394.25, -74.0463) -> (396.25, -72.8916)
  line L2417 (363.25, -106.5822) -> (361.25, -105.4275)
  line L2418 (359.25, -99.8916) -> (361.25, -101.0463)
  line L2419 (361.25, -96.4275) -> (359.25, -97.5822)
  line L2420 (392.25, -90.8916) -> (394.25, -92.0463)
  line L2421 (344.75, -92.0463) -> (346.75, -90.8916)
  line L2422 (370.25, -88.5822) -> (370.25, -90.8916)
  line L2423 (347.5, -96.8094) -> (349.5, -95.6547)
  line L2424 (344.75, -78.4275) -> (342.75, -79.5822)
  line L2425 (391.5, -87.8094) -> (393.5, -86.6547)
  line L2426 (347.5, -96.8094) -> (349.5, -95.6547)
  line L2427 (392.25, -54.8916) -> (394.25, -56.0463)
  line L2428 (392.25, -72.8916) -> (394.25, -74.0463)
  line L2429 (394.25, -78.4275) -> (392.25, -79.5822)
  line L2430 (347.5, -92.1906) -> (345.5, -93.3453)
  line L2431 (349.5, -93.3453) -> (347.5, -92.1906)
  line L2432 (374.25, -90.8916) -> (374.25, -88.5822)
  line L2433 (344.75, -60.4275) -> (343.5641, -61.1121)
  line L2434 (392.25, -90.8916) -> (394.25, -92.0463)
  line L2435 (342.75, -81.8916) -> (344.75, -83.0463)
  line L2436 (342.75, -72.8916) -> (344.75, -74.0463)
  line L2437 (344.75, -87.4275) -> (342.75, -88.5822)
  line L2438 (401.75, -72.8916) -> (401.75, -70.5822)
  line L2439 (393.5, -84.3453) -> (391.5, -83.1906)
  line L2440 (344.75, -69.4275) -> (342.75, -70.5822)
  line L2441 (397, -69.8094) -> (399, -68.6547)
  line L2442 (399.75, -69.4275) -> (397.75, -70.5822)
  line L2443 (397.75, -70.5822) -> (397.75, -72.8916)
  line L2444 (391.5, -60.8094) -> (393.5, -59.6547)
  line L2445 (345.8335, -95.8473) -> (347.5, -96.8094)
  line L2446 (345.8335, -95.8473) -> (347.5, -96.8094)
  line L2447 (391.5, -51.8094) -> (393.5, -50.6547)
  line L2448 (391.5, -69.8094) -> (393.5, -68.6547)
  line L2449 (399.75, -74.0463) -> (401.75, -72.8916)
  line L2450 (391.5, -69.8094) -> (393.5, -68.6547)
  line L2451 (392.25, -72.8916) -> (394.25, -74.0463)
  line L2452 (342.75, -63.8916) -> (344.75, -65.0463)
  line L2453 (396.25, -70.5822) -> (394.25, -69.4275)
  line L2454 (393.5, -93.3453) -> (391.5, -92.1906)
  line L2455 (342.75, -81.8916) -> (344.75, -83.0463)
  line L2456 (347.5, -92.1906) -> (345.5, -93.3453)
  line L2457 (397, -74.1906) -> (395, -75.3453)
  line L2458 (397.75, -72.8916) -> (399.75, -74.0463)
  line L2459 (396.25, -70.5822) -> (394.25, -69.4275)
  line L2460 (391.5, -60.8094) -> (393.5, -59.6547)
  line L2461 (344.75, -78.4275) -> (342.75, -79.5822)
  line L2462 (397.75, -72.8916) -> (399.75, -74.0463)
  line L2463 (344.75, -87.4275) -> (342.75, -88.5822)
  line L2464 (394.25, -74.0463) -> (396.25, -72.8916)
  line L2465 (344.75, -69.4275) -> (342.75, -70.5822)
  line L2466 (349.5, -93.3453) -> (347.5, -92.1906)
  line L2467 (342.75, -63.8916) -> (344.75, -65.0463)
  line L2468 (393.5, -84.3453) -> (391.5, -83.1906)
  line L2469 (395, -68.6547) -> (397, -69.8094)
  line L2470 (394.25, -51.4275) -> (392.25, -52.5822)
  line L2471 (401.75, -72.8916) -> (401.75, -70.5822)
  line L2472 (393.5, -48.3453) -> (391.5, -47.1906)
  line L2473 (393.5, -77.6547) -> (393.5, -75.3453)
  line L2474 (399, -77.6547) -> (399, -75.3453)
  line L2475 (363.25, -79.5822) -> (361.25, -78.4275)
  line L2476 (370.25, -106.5822) -> (370.25, -108.8916)
  line L2477 (399.75, -74.0463) -> (401.75, -72.8916)
  line L2478 (374.25, -88.5822) -> (372.25, -87.4275)
  line L2479 (341.8476, -87.7214) -> (342, -87.8094)
  line L2480 (361.25, -105.4275) -> (359.25, -106.5822)
  line L2481 (361.25, -92.0463) -> (363.25, -90.8916)
  line L2482 (363.25, -106.5822) -> (361.25, -105.4275)
  line L2483 (343.2193, -91.1625) -> (344.75, -92.0463)
  line L2484 (393.5, -77.6547) -> (393.5, -75.3453)
  line L2485 (361.25, -101.0463) -> (363.25, -99.8916)
  line L2486 (374.25, -106.5822) -> (372.25, -105.4275)
  line L2487 (361.25, -47.0463) -> (363.25, -45.8916)
  line L2488 (399, -77.6547) -> (399, -75.3453)
  line L2489 (361.25, -83.0463) -> (363.25, -81.8916)
  line L2490 (345.5, -93.3453) -> (345.5, -95.3348)
  arc A79 (345.5, -95.3348) -> (345.8335, -95.8473) centre (375, -76.5) ccw
  line L2491 (341.25, -72.8916) -> (341.25, -70.5822)
  line L2492 (373, -111.3453) -> (373, -111.4428)
  line L2493 (395, -75.3453) -> (395, -77.6547)
  line L2494 (370.25, -106.5822) -> (370.25, -108.8916)
  line L2495 (343.2193, -91.1625) -> (344.75, -92.0463)
  line L2496 (372.25, -105.4275) -> (370.25, -106.5822)
  line L2497 (400.5, -77.6547) -> (402.5, -78.8094)
  line L2498 (344.75, -92.0463) -> (346.75, -90.8916)
  line L2499 (345.5, -93.3453) -> (345.5, -95.3348)
  line L2500 (397, -69.8094) -> (399, -68.6547)
  line L2501 (342.75, -72.8916) -> (344.75, -74.0463)
  line L2502 (394.25, -87.4275) -> (392.25, -88.5822)
  line L2503 (373, -104.6547) -> (375, -105.8094)
  line L2504 (341.25, -72.8916) -> (341.25, -70.5822)
  line L2505 (375, -110.1906) -> (373, -111.3453)
  line L2506 (400.5, -75.3453) -> (400.5, -77.6547)
  line L2507 (402.5, -83.1906) -> (400.5, -84.3453)
  line L2508 (342.75, -70.5822) -> (342.75, -72.8916)
  line L2509 (392.25, -99.8916) -> (394.25, -101.0463)
  line L2510 (373, -104.6547) -> (375, -105.8094)
  line L2511 (344.75, -60.4275) -> (343.5641, -61.1121)
  line L2512 (395, -75.3453) -> (395, -77.6547)
  arc A80 (340.5732, -70.1914) -> (340.1253, -73.5409) centre (375, -76.5) ccw
  line L2513 (361.25, -96.4275) -> (359.25, -97.5822)
  line L2514 (400.5, -68.6547) -> (402.5, -69.8094)
  line L2515 (394.25, -69.4275) -> (392.25, -70.5822)
  line L2516 (371.5, -84.3453) -> (369.5, -83.1906)
  line L2517 (363.25, -97.5822) -> (361.25, -96.4275)
  line L2518 (394.25, -87.4275) -> (392.25, -88.5822)
  line L2519 (393.5, -48.3453) -> (391.5, -47.1906)
  line L2520 (399.75, -69.4275) -> (397.75, -70.5822)
  line L2521 (342.75, -70.5822) -> (342.75, -72.8916)
  line L2522 (393.5, -75.3453) -> (391.5, -74.1906)
  arc A81 (345.5, -95.3348) -> (345.8335, -95.8473) centre (375, -76.5) ccw
  line L2523 (400.5, -75.3453) -> (400.5, -77.6547)
  line L2524 (394.25, -69.4275) -> (392.25, -70.5822)
  arc A82 (340.5732, -70.1914) -> (340.1253, -73.5409) centre (375, -76.5) ccw
  line L2525 (361.25, -56.0463) -> (363.25, -54.8916)
  arc A83 (359.25, -107.756) -> (362.6388, -109.2445) centre (375, -76.5) ccw
  line L2526 (342, -83.1906) -> (340.789, -83.8898)
  line L2527 (404.5, -84.3453) -> (402.5, -83.1906)
  line L2528 (394.25, -60.4275) -> (392.25, -61.5822)
  line L2529 (344, -84.3453) -> (342, -83.1906)
  line L2530 (342, -69.8094) -> (344, -68.6547)
  line L2531 (341.8476, -87.7214) -> (342, -87.8094)
  line L2532 (363.25, -88.5822) -> (361.25, -87.4275)
  line L2533 (342, -87.8094) -> (344, -86.6547)
  line L2534 (402.5, -78.8094) -> (404.5, -77.6547)
  line L2535 (402.5, -69.8094) -> (404.5, -68.6547)
  line L2536 (374.25, -88.5822) -> (372.25, -87.4275)
  line L2537 (372.25, -110.0463) -> (374.25, -108.8916)
  line L2538 (370.25, -108.8916) -> (372.25, -110.0463)
  line L2539 (340.4891, -82.3309) -> (341.25, -81.8916)
  line L2540 (342.75, -88.5822) -> (342.75, -90.0992)
  line L2541 (375, -110.1906) -> (373, -111.3453)
  line L2542 (362, -59.6547) -> (364, -60.8094)
  line L2543 (342, -83.1906) -> (340.789, -83.8898)
  line L2544 (402.5, -83.1906) -> (400.5, -84.3453)
  line L2545 (341.25, -70.5822) -> (340.5732, -70.1914)
  line L2546 (371.5, -84.3453) -> (369.5, -83.1906)
  line L2547 (342.75, -62.9008) -> (342.75, -63.8916)
  line L2548 (342, -87.8094) -> (344, -86.6547)
  line L2549 (402.5, -78.8094) -> (404.5, -77.6547)
  line L2550 (372.25, -105.4275) -> (370.25, -106.5822)
  line L2551 (392.25, -63.8916) -> (394.25, -65.0463)
  line L2552 (370.25, -81.8916) -> (372.25, -83.0463)
  line L2553 (370.25, -81.8916) -> (372.25, -83.0463)
  arc A84 (343.5641, -61.1121) -> (342.75, -62.9008) centre (375, -76.5) ccw
  line L2554 (363.25, -52.5822) -> (361.25, -51.4275)
  line L2555 (404.5, -75.3453) -> (402.5, -74.1906)
  line L2556 (373, -86.6547) -> (375, -87.8094)
  line L2557 (372.25, -110.0463) -> (374.25, -108.8916)
  line L2558 (370.25, -108.8916) -> (372.25, -110.0463)
  line L2559 (402.5, -74.1906) -> (400.5, -75.3453)
  line L2560 (361.25, -105.4275) -> (359.25, -106.5822)
  line L2561 (344, -68.6547) -> (344, -66.3453)
  arc A85 (343.5641, -61.1121) -> (342.75, -62.9008) centre (375, -76.5) ccw
  line L2562 (402.5, -69.8094) -> (404.5, -68.6547)
  line L2563 (342.75, -62.9008) -> (342.75, -63.8916)
  line L2564 (371.5, -86.6547) -> (371.5, -84.3453)
  line L2565 (359.25, -90.8916) -> (361.25, -92.0463)
  line L2566 (402.5, -74.1906) -> (400.5, -75.3453)
  line L2567 (372.25, -83.0463) -> (374.25, -81.8916)
  line L2568 (340.789, -69.1102) -> (342, -69.8094)
  arc A86 (340.789, -83.8898) -> (341.8476, -87.7214) centre (375, -76.5) ccw
  line L2569 (374.25, -106.5822) -> (372.25, -105.4275)
  line L2570 (340.4891, -82.3309) -> (341.25, -81.8916)
  line L2571 (393.5, -93.3453) -> (391.5, -92.1906)
  line L2572 (373, -111.3453) -> (373, -111.4428)
  line L2573 (373, -86.6547) -> (375, -87.8094)
  line L2574 (342, -69.8094) -> (344, -68.6547)
  line L2575 (400.5, -68.6547) -> (402.5, -69.8094)
  line L2576 (374.25, -108.8916) -> (374.25, -106.5822)
  line L2577 (371.5, -86.6547) -> (371.5, -84.3453)
  line L2578 (392.25, -54.8916) -> (394.25, -56.0463)
  line L2579 (391.5, -96.8094) -> (393.5, -95.6547)
  line L2580 (404.5, -75.3453) -> (402.5, -74.1906)
  line L2581 (372.25, -83.0463) -> (374.25, -81.8916)
  line L2582 (344, -68.6547) -> (344, -66.3453)
  line L2583 (374.25, -108.8916) -> (374.25, -106.5822)
  line L2584 (400.5, -77.6547) -> (402.5, -78.8094)
  line L2585 (369.5, -87.8094) -> (371.5, -86.6547)
  line L2586 (342.75, -88.5822) -> (342.75, -90.0992)
  line L2587 (344, -66.3453) -> (342, -65.1906)
  line L2588 (344, -86.6547) -> (344, -84.3453)
  line L2589 (391.5, -96.8094) -> (393.5, -95.6547)
  line L2590 (372.25, -87.4275) -> (370.25, -88.5822)
  line L2591 (375, -83.1906) -> (373, -84.3453)
  line L2592 (404.5, -84.3453) -> (402.5, -83.1906)
  line L2593 (364, -74.1906) -> (362, -75.3453)
  line L2594 (344, -86.6547) -> (344, -84.3453)
  line L2595 (344, -66.3453) -> (342, -65.1906)
  line L2596 (404.5, -86.6547) -> (404.5, -84.3453)
  line L2597 (353, -56.1906) -> (351, -57.3453)
  line L2598 (350.25, -65.0463) -> (352.25, -63.8916)
  line L2599 (363.25, -45.8916) -> (363.25, -43.5822)
  line L2600 (360.5, -50.6547) -> (360.5, -48.3453)
  line L2601 (383.25, -60.4275) -> (381.25, -61.5822)
  line L2602 (352.25, -63.8916) -> (352.25, -61.5822)
  line L2603 (346.75, -70.5822) -> (344.75, -69.4275)
  line L2604 (364.75, -45.8916) -> (366.75, -47.0463)
  line L2605 (356.5, -50.6547) -> (358.5, -51.8094)
  line L2606 (353, -69.8094) -> (355, -68.6547)
  line L2607 (380.5, -56.1906) -> (378.5, -57.3453)
  line L2608 (357.75, -52.5822) -> (355.75, -51.4275)
  line L2609 (352.25, -63.8916) -> (352.25, -61.5822)
  line L2610 (381.25, -54.8916) -> (383.25, -56.0463)
  line L2611 (364.75, -43.5822) -> (364.75, -45.8916)
  line L2612 (359.25, -45.8916) -> (361.25, -47.0463)
  line L2613 (366, -48.3453) -> (364, -47.1906)
  line L2614 (344.75, -65.0463) -> (346.75, -63.8916)
  line L2615 (347.5, -69.8094) -> (349.5, -68.6547)
  line L2616 (346.75, -63.8916) -> (346.75, -61.5822)
  line L2617 (383.25, -56.0463) -> (385.25, -54.8916)
  line L2618 (369.5, -47.1906) -> (367.5, -48.3453)
  line L2619 (363.25, -43.5822) -> (363.1955, -43.5507)
  line L2620 (358.5, -47.1906) -> (356.5, -48.3453)
  line L2621 (348.25, -63.8916) -> (350.25, -65.0463)
  line L2622 (366.573, -42.5296) -> (364.75, -43.5822)
  line L2623 (381.25, -54.8916) -> (383.25, -56.0463)
  line L2624 (353, -65.1906) -> (351, -66.3453)
  line L2625 (368.75, -43.5822) -> (366.8218, -42.4689)
  line L2626 (366.75, -47.0463) -> (368.75, -45.8916)
  line L2627 (378.5, -59.6547) -> (380.5, -60.8094)
  line L2628 (378.5, -59.6547) -> (380.5, -60.8094)
  line L2629 (353, -51.8094) -> (355, -50.6547)
  line L2630 (368.75, -45.8916) -> (368.75, -43.5822)
  line L2631 (346.75, -63.8916) -> (346.75, -61.5822)
  line L2632 (359.25, -45.8916) -> (361.25, -47.0463)
  line L2633 (355, -50.6547) -> (355, -48.3453)
  line L2634 (360.5, -50.6547) -> (360.5, -48.3453)
  line L2635 (383.25, -60.4275) -> (381.25, -61.5822)
  line L2636 (364.75, -45.8916) -> (366.75, -47.0463)
  line L2637 (352.25, -52.5822) -> (350.4572, -51.5471)
  line L2638 (355, -50.6547) -> (355, -48.3453)
  line L2639 (363.25, -45.8916) -> (363.25, -43.5822)
  line L2640 (366.573, -42.5296) -> (364.75, -43.5822)
  line L2641 (385.25, -61.5822) -> (383.25, -60.4275)
  line L2642 (375.75, -54.8916) -> (377.75, -56.0463)
  line L2643 (348.25, -61.5822) -> (348.25, -63.8916)
  line L2644 (362, -48.3453) -> (362, -50.6547)
  line L2645 (352.25, -52.5822) -> (350.4572, -51.5471)
  line L2646 (362, -48.3453) -> (362, -50.6547)
  line L2647 (355, -66.3453) -> (353, -65.1906)
  line L2648 (347.5, -65.1906) -> (345.5, -66.3453)
  arc A87 (350.4572, -51.5471) -> (348.25, -53.9293) centre (375, -76.5) ccw
  line L2649 (348.25, -61.5822) -> (348.25, -63.8916)
  line L2650 (366.75, -47.0463) -> (368.75, -45.8916)
  line L2651 (345.5, -66.3453) -> (345.5, -68.6547)
  line L2652 (345.5, -66.3453) -> (345.5, -68.6547)
  line L2653 (347.5, -56.1906) -> (345.8335, -57.1527)
  line L2654 (350.25, -56.0463) -> (352.25, -54.8916)
  line L2655 (355, -48.3453) -> (354.558, -48.0901)
  line L2656 (352.25, -61.5822) -> (350.25, -60.4275)
  line L2657 (344.75, -65.0463) -> (346.75, -63.8916)
  arc A88 (345.8335, -57.1527) -> (345.5, -57.6652) centre (375, -76.5) ccw
  line L2658 (350.25, -60.4275) -> (348.25, -61.5822)
  line L2659 (358.5, -47.1906) -> (356.5, -48.3453)
  line L2660 (349.5, -57.3453) -> (347.5, -56.1906)
  line L2661 (349.5, -68.6547) -> (349.5, -66.3453)
  line L2662 (360.5, -48.3453) -> (358.5, -47.1906)
  line L2663 (353, -56.1906) -> (351, -57.3453)
  line L2664 (349.5, -57.3453) -> (347.5, -56.1906)
  line L2665 (350.25, -69.4275) -> (348.25, -70.5822)
  line L2666 (345.5, -68.6547) -> (347.5, -69.8094)
  line L2667 (345.5, -57.6652) -> (345.5, -59.6547)
  line L2668 (346.75, -61.5822) -> (344.75, -60.4275)
  line L2669 (346.75, -61.5822) -> (344.75, -60.4275)
  line L2670 (366, -48.3453) -> (364, -47.1906)
  line L2671 (345.5, -68.6547) -> (347.5, -69.8094)
  line L2672 (347.5, -69.8094) -> (349.5, -68.6547)
  line L2673 (356.5, -48.3453) -> (356.5, -50.6547)
  line L2674 (348.25, -54.8916) -> (350.25, -56.0463)
  line L2675 (351, -66.3453) -> (351, -68.6547)
  line L2676 (358.5, -51.8094) -> (360.5, -50.6547)
  line L2677 (348.25, -54.8916) -> (350.25, -56.0463)
  arc A89 (354.558, -48.0901) -> (351.2448, -50.7961) centre (375, -76.5) ccw
  line L2678 (360.5, -48.3453) -> (358.5, -47.1906)
  line L2679 (349.5, -59.6547) -> (349.5, -57.3453)
  arc A90 (366.8218, -42.4689) -> (366.573, -42.5296) centre (375, -76.5) ccw
  line L2680 (350.25, -65.0463) -> (352.25, -63.8916)
  line L2681 (349.5, -68.6547) -> (349.5, -66.3453)
  line L2682 (355.75, -51.4275) -> (353.75, -52.5822)
  line L2683 (350.25, -69.4275) -> (348.25, -70.5822)
  line L2684 (345.5, -57.6652) -> (345.5, -59.6547)
  line L2685 (347.5, -65.1906) -> (345.5, -66.3453)
  line L2686 (353, -51.8094) -> (355, -50.6547)
  line L2687 (368.3398, -42.1395) -> (369.5, -42.8094)
  line L2688 (349.5, -66.3453) -> (347.5, -65.1906)
  line L2689 (358.5, -51.8094) -> (360.5, -50.6547)
  line L2690 (351, -57.3453) -> (351, -59.6547)
  line L2691 (352.25, -70.5822) -> (350.25, -69.4275)
  line L2692 (351, -68.6547) -> (353, -69.8094)
  line L2693 (368.75, -43.5822) -> (366.8218, -42.4689)
  line L2694 (351, -68.6547) -> (353, -69.8094)
  line L2695 (347.5, -56.1906) -> (345.8335, -57.1527)
  line L2696 (351, -59.6547) -> (353, -60.8094)
  line L2697 (355.75, -51.4275) -> (353.75, -52.5822)
  line L2698 (347.5, -60.8094) -> (349.5, -59.6547)
  arc A91 (345.8335, -57.1527) -> (345.5, -57.6652) centre (375, -76.5) ccw
  line L2699 (345.5, -59.6547) -> (347.5, -60.8094)
  line L2700 (351.2448, -50.7961) -> (353, -51.8094)
  line L2701 (369.5, -47.1906) -> (367.5, -48.3453)
  line L2702 (351.2448, -50.7961) -> (353, -51.8094)
  line L2703 (361.25, -51.4275) -> (359.25, -52.5822)
  arc A92 (366.8218, -42.4689) -> (366.573, -42.5296) centre (375, -76.5) ccw
  line L2704 (351, -57.3453) -> (351, -59.6547)
  line L2705 (350.25, -60.4275) -> (348.25, -61.5822)
  line L2706 (349.5, -66.3453) -> (347.5, -65.1906)
  line L2707 (352.25, -61.5822) -> (350.25, -60.4275)
  line L2708 (345.5, -59.6547) -> (347.5, -60.8094)
  line L2709 (350.25, -56.0463) -> (352.25, -54.8916)
  line L2710 (351, -59.6547) -> (353, -60.8094)
  line L2711 (347.5, -60.8094) -> (349.5, -59.6547)
  line L2712 (349.5, -59.6547) -> (349.5, -57.3453)
  line L2713 (388, -75.3453) -> (386, -74.1906)
  line L2714 (353.75, -79.5822) -> (353.75, -81.8916)
  line L2715 (383.25, -65.0463) -> (385.25, -63.8916)
  line L2716 (383.25, -69.4275) -> (381.25, -70.5822)
  line L2717 (378.5, -84.3453) -> (378.5, -86.6547)
  line L2718 (353.75, -72.8916) -> (355.75, -74.0463)
  line L2719 (388.75, -47.0463) -> (390.75, -45.8916)
  line L2720 (384, -50.6547) -> (386, -51.8094)
  line L2721 (389.5, -77.6547) -> (391.5, -78.8094)
  line L2722 (384, -48.3453) -> (384, -50.6547)
  line L2723 (384, -77.6547) -> (386, -78.8094)
  line L2724 (382.5, -86.6547) -> (382.5, -84.3453)
  line L2725 (388.75, -78.4275) -> (386.75, -79.5822)
  line L2726 (380.5, -87.8094) -> (382.5, -86.6547)
  line L2727 (385.25, -70.5822) -> (383.25, -69.4275)
  line L2728 (386.75, -79.5822) -> (386.75, -81.8916)
  line L2729 (377.75, -87.4275) -> (375.75, -88.5822)
  line L2730 (359.25, -79.5822) -> (359.25, -81.8916)
  line L2731 (357.75, -81.8916) -> (357.75, -79.5822)
  line L2732 (383.25, -65.0463) -> (385.25, -63.8916)
  line L2733 (385.25, -70.5822) -> (383.25, -69.4275)
  line L2734 (353.75, -79.5822) -> (353.75, -81.8916)
  line L2735 (388, -50.6547) -> (388, -48.3453)
  line L2736 (360.5, -68.6547) -> (360.5, -66.3453)
  line L2737 (389.5, -50.6547) -> (391.5, -51.8094)
  line L2738 (386.75, -43.5822) -> (386.75, -45.8916)
  line L2739 (381.25, -63.8916) -> (383.25, -65.0463)
  line L2740 (392.25, -61.5822) -> (392.25, -63.8916)
  line L2741 (375.75, -81.8916) -> (377.75, -83.0463)
  line L2742 (359.25, -79.5822) -> (359.25, -81.8916)
  line L2743 (358.5, -69.8094) -> (360.5, -68.6547)
  line L2744 (388, -48.3453) -> (386, -47.1906)
  line L2745 (377.75, -83.0463) -> (379.75, -81.8916)
  line L2746 (379.75, -88.5822) -> (377.75, -87.4275)
  line L2747 (386, -74.1906) -> (384, -75.3453)
  line L2748 (391.5, -74.1906) -> (389.5, -75.3453)
  line L2749 (388, -77.6547) -> (388, -75.3453)
  line L2750 (385.25, -81.8916) -> (385.25, -79.5822)
  line L2751 (388, -77.6547) -> (388, -75.3453)
  line L2752 (386.75, -45.8916) -> (388.75, -47.0463)
  line L2753 (383.25, -69.4275) -> (381.25, -70.5822)
  line L2754 (353.75, -63.8916) -> (355.75, -65.0463)
  line L2755 (377, -86.6547) -> (377, -84.3453)
  line L2756 (379.75, -45.8916) -> (379.75, -43.5822)
  line L2757 (357.75, -81.8916) -> (357.75, -79.5822)
  line L2758 (355.75, -65.0463) -> (357.75, -63.8916)
  line L2759 (358.5, -65.1906) -> (356.5, -66.3453)
  line L2760 (371.5, -48.3453) -> (369.5, -47.1906)
  line L2761 (386, -78.8094) -> (388, -77.6547)
  line L2762 (378.5, -86.6547) -> (380.5, -87.8094)
  line L2763 (380.5, -83.1906) -> (378.5, -84.3453)
  line L2764 (384, -50.6547) -> (386, -51.8094)
  line L2765 (355, -68.6547) -> (355, -66.3453)
  line L2766 (378.5, -66.3453) -> (378.5, -68.6547)
  line L2767 (352.25, -54.8916) -> (352.25, -52.5822)
  line L2768 (360.5, -66.3453) -> (358.5, -65.1906)
  line L2769 (381.25, -63.8916) -> (383.25, -65.0463)
  line L2770 (388, -50.6547) -> (388, -48.3453)
  line L2771 (386, -51.8094) -> (388, -50.6547)
  line L2772 (386, -74.1906) -> (384, -75.3453)
  line L2773 (355.75, -69.4275) -> (353.75, -70.5822)
  line L2774 (366.75, -74.0463) -> (368.75, -72.8916)
  line L2775 (386.75, -79.5822) -> (386.75, -81.8916)
  line L2776 (380.5, -87.8094) -> (382.5, -86.6547)
  line L2777 (384, -75.3453) -> (384, -77.6547)
  line L2778 (388.75, -78.4275) -> (386.75, -79.5822)
  line L2779 (347.5, -87.8094) -> (349.5, -86.6547)
  line L2780 (380.5, -74.1906) -> (378.5, -75.3453)
  line L2781 (389.5, -57.3453) -> (389.5, -59.6547)
  line L2782 (380.5, -83.1906) -> (378.5, -84.3453)
  line L2783 (366, -77.6547) -> (366, -75.3453)
  line L2784 (391.5, -74.1906) -> (389.5, -75.3453)
  line L2785 (390.75, -63.8916) -> (390.75, -61.5822)
  line L2786 (384, -48.3453) -> (384, -50.6547)
  line L2787 (386, -47.1906) -> (384, -48.3453)
  line L2788 (375.75, -61.5822) -> (375.75, -63.8916)
  line L2789 (353, -87.8094) -> (355, -86.6547)
  line L2790 (355.75, -69.4275) -> (353.75, -70.5822)
  line L2791 (358.5, -65.1906) -> (356.5, -66.3453)
  line L2792 (366.75, -78.4275) -> (364.75, -79.5822)
  line L2793 (355, -84.3453) -> (353, -83.1906)
  line L2794 (388.75, -47.0463) -> (390.75, -45.8916)
  line L2795 (385.25, -45.8916) -> (385.25, -43.5822)
  line L2796 (369.5, -69.8094) -> (371.5, -68.6547)
  line L2797 (386, -51.8094) -> (388, -50.6547)
  line L2798 (391.5, -47.1906) -> (389.5, -48.3453)
  line L2799 (353.75, -52.5822) -> (353.75, -54.8916)
  line L2800 (390.75, -52.5822) -> (388.75, -51.4275)
  line L2801 (358.5, -69.8094) -> (360.5, -68.6547)
  line L2802 (356.5, -66.3453) -> (356.5, -68.6547)
  line L2803 (355, -68.6547) -> (355, -66.3453)